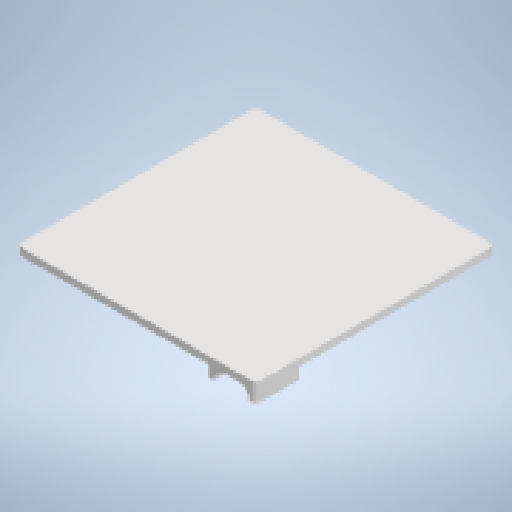
# Autodesk Inventor part: plateauMoteur6G
Saved by Autodesk Inventor 2025.2 (Build 292293000, 293)
## iProperties
Created: 2025-02-16
Part Number: plateauMoteur6G
Material: Générique
Document SubType Name: Modeling
Designer: arthu
Density: 1 g/cm^3
Appearance: Par défaut
Author: arthu
Autodesk Inventor part; units mm, degrees
ref_plane "YZ Plane" through (0, 0, 0) normal (1, 0, 0) x (0, 1, 0)
ref_plane "XZ Plane" through (0, 0, 0) normal (0, 1, 0) x (-1, 0, 0)
ref_plane "XY Plane" through (0, 0, 0) normal (0, 0, 1) x (1, 0, 0)
sketch "Esquisse1" plane through (0, 0, 0) normal (0, 1, 0) x (-1, 0, 0)
  line L0 (0, 0) -> (100, 0)
  line L1 (100, 0) -> (100, -100)
  line L2 (100, -100) -> (0, -100)
  line L3 (0, -100) -> (0, 0)
  dimension "d0" = 100
  dimension "d1" = 100
  constraints: 8 end point, 2 parallel, 1 horizontal, 1 perpendicular
  measures "d0" distance of L1.end L2.end
  measures "d1" distance of L0.end L1.end
extrude "Extrusion1" add sketch "Esquisse1" along normal blind 3
fillet "Congé1" radius 2 4 edges at (0, 1.5, 0) (-100, 1.5, 0) (-100, 1.5, -100) (0, 1.5, -100)
sketch "Esquisse9" plane through (0, 0, 0) normal (0, -1, 0) x (1, 0, 0)
  line L0 (0, 0) -> (-20, 0)
  line L1 (-20, 0) -> (-20, -100)
  line L2 (-20, -100) -> (0, -100)
  line L3 (0, -100) -> (0, 0)
  dimension "d117" = 20
  dimension "d118" = 100
  constraints: 8 end point, 2 parallel, 1 horizontal, 1 perpendicular
  measures "d117" distance of L2.end L1.end
  measures "d118" distance of L1.end L0.end
extrude "Extrusion5" add sketch "Esquisse9" along normal blind 4.7
sketch "Esquisse10" plane through (-98, 3, 0) normal (0, 0, 1) x (1, 0, 0)
  line L0 (78, -7.7) -> (98, -7.7) projected
  line L1 (87.7, -3) -> (90.8, -3)
  line L2 (87.7, -3) -> (85.2, -3)
  line L3 (78, -3) -> (98, -3) projected
  arc A0 (85.2, -3) -> (80.5, -7.7) centre (85.2, -7.7) ccw
  arc A1 (95.5, -7.7) -> (90.8, -3) centre (90.8, -7.7) ccw
  point P0 (93.3, -3)
  dimension "d123" = 9.4
  constraints: 6 end point, 6 point on line, 4 point on circle, 2 centre point, 1 horizontal
  measures "d123" diameter of A0
extrude "Extrusion6" cut sketch "Esquisse10" against normal blind 100
sketch "Esquisse11" plane through (-98, 3, 0) normal (0, 0, 1) x (1, 0, 0)
  line L0 (-2, 0) -> (-2, -3) projected
  line L1 (-2, -3) -> (18, -3)
  line L2 (18, -3) -> (18, -7.7)
  line L3 (18, -7.7) -> (-2, -7.7)
  line L4 (-2, -7.7) -> (-2, -3)
  arc A0 (5.2, -3) -> (0.5, -7.7) centre (5.2, -7.7) ccw
  arc A1 (15.5, -7.7) -> (10.8, -3) centre (10.8, -7.7) ccw
  line L5 (10.8, -3) -> (5.2, -3)
  line L6 (0, -3) -> (78, -3) projected
  point P0 (98, -3)
  dimension "d132" = 20
  dimension "d133" = 9.4
  dimension "d134" = 9.4
  constraints: 10 end point, 6 point on line, 4 point on circle, 2 centre point, 2 parallel, 1 collinear, 1 horizontal, 1 perpendicular, 1 tangent
  measures "d132" distance of L2.end L3.end
  measures "d133" diameter of A0
  measures "d134" diameter of A1
extrude "Extrusion7" add sketch "Esquisse11" against normal blind 100 contours L1 A0 L3 L4 | L1 L2 L3 A1
fillet "Congé4" radius 2 4 edges at (0, -2.35, 0) (0, -2.35, -100) (-100, -2.35, 0) (-100, -2.35, -100)
sketch "Esquisse12" plane through (-100, 3, -98) normal (-1, 0, 0) x (0, 0, 1)
  line L0 (80, -3) -> (16, -3)
  line L1 (16, -3) -> (16, -7.7)
  line L2 (16, -7.7) -> (80, -7.7)
  line L3 (80, -7.7) -> (80, -3)
  point P0 (98, -3)
  dimension "d138" = 64
  dimension "d139" = 4.7
  constraints: 8 end point, 2 parallel, 1 horizontal, 1 perpendicular
  measures "d138" distance of L2.end L1.end
  measures "d139" distance of L1.end L0.end
extrude "Extrusion8" cut sketch "Esquisse12" against normal blind 100
